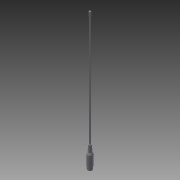
# Autodesk Inventor part: nagoya771
Saved by Autodesk Inventor 2014 (Build 180170000, 170)
## iProperties
Created: 2015-02-27
Part Number: nagoya771
Material: Generic
Document SubType Name: Modeling
Designer: Admin
Density: 1 g/cm^3
Appearance: Default
Author: Admin
Autodesk Inventor part; units mm, degrees
ref_plane "YZ Plane" through (0, 0, 0) normal (1, 0, 0) x (0, 1, 0)
ref_plane "XZ Plane" through (0, 0, 0) normal (0, 1, 0) x (-1, 0, 0)
ref_plane "XY Plane" through (0, 0, 0) normal (0, 0, 1) x (1, 0, 0)
sketch "Boceto1" plane through (0, 0, 0) normal (0, 0, 1) x (1, 0, 0)
  circle A0 centre (0, 0) radius 6.5
  dimension "d0" = 13
  constraints: 1 centre point, 1 coincident
  measures "d0" diameter of A0
extrude "Extrusión1" add sketch "Boceto1" along normal blind 8.25
sketch "Boceto2" plane through (0, 0, 8.25) normal (0, 0, 1) x (1, 0, 0)
  circle A0 centre (0, 0) radius 6.5 projected
  circle A1 centre (0, 0) radius 7.35
  dimension "d3" = 14.7
  constraints: 1 centre point, 1 coincident
  measures "d3" diameter of A1
extrude "Extrusión2" add sketch "Boceto2" along normal blind 29.75 contours A0 | A1
sketch "Boceto3" plane through (0, 0, 38) normal (0, 0, 1) x (1, 0, 0)
  circle A0 centre (0, 0) radius 7.35 projected
  circle A1 centre (0, 0) radius 5.65
  dimension "d6" = 11.3
  constraints: 1 centre point, 1 coincident
  measures "d6" diameter of A1
extrude "Extrusión3" add sketch "Boceto3" along normal blind 4.7 contours A1
sketch "Boceto4" plane through (0, 0, 0) normal (1, 0, 0) x (0, 1, 0)
  line L0 (5.65, 42.7) -> (-5.65, 42.7) projected
  line L1 (7.35, 38) -> (-7.35, 38) projected
  line L2 (5.65, 42.7) -> (7.35, 38)
  line L3 (5.65, 38) -> (5.65, 42.7)
  line L4 (0, 42.7) -> (0, 50.6655) construction
  point P0 (0, 0)
  constraints: 6 end point, 1 midpoint, 1 parallel, 1 perpendicular, 1 point on line
revolve "Revolución1" add sketch "Boceto4" angle 360 about axis through (0, 0, 42.7) along (0, 0, 1)
sketch "Boceto7" plane through (0, 0, 0) normal (1, 0, 0) x (0, 1, 0)
  line L0 (5.65, 42.7) -> (-5.65, 42.7) projected
  line L1 (0, 42.7) -> (4.95, 42.7) construction
  line L2 (0, 42.7) -> (0, 62.2)
  line L3 (0, 62.2) -> (3.9, 62.2)
  line L4 (3.9, 62.2) -> (4.95, 42.7)
  point P0 (0, 0)
  dimension "d13" = 4.95
  dimension "d14" = 19.5
  dimension "d15" = 3.9
  constraints: 8 end point, 2 perpendicular, 1 midpoint, 1 point on line
  measures "d13" distance of L1.start L1.end
  measures "d14" distance of L1.start L2.end
  measures "d15" distance of L2.end L3.end
revolve "Revolución2" add sketch "Boceto7" angle 360 about axis through (0, 0, 42.7) along (0, 0, 1)
sketch "Boceto8" plane through (0, 0, 62.2) normal (0, 0, 1) x (1, 0, 0)
  circle A0 centre (0, 0) radius 3.9 projected
  circle A1 centre (0, 0) radius 2.15
  dimension "d17" = 4.3
  constraints: 1 centre point, 1 coincident
  measures "d17" diameter of A1
extrude "Extrusión5" add sketch "Boceto8" along normal blind 82 contours A1
sketch "Boceto9" plane through (0, 0, 144.2) normal (0, 0, 1) x (1, 0, 0)
  circle A0 centre (0, 0) radius 2.15 projected
  circle A1 centre (0, 0) radius 1.95
  dimension "d20" = 3.9
  constraints: 1 centre point, 1 coincident
  measures "d20" diameter of A1
extrude "Extrusión6" add sketch "Boceto9" along normal blind 238 contours A1
sketch "Boceto10" plane through (0, 0, 382.2) normal (0, 0, 1) x (1, 0, 0)
  circle A0 centre (0, 0) radius 1.95 projected
  circle A1 centre (0, 0) radius 2.9
  dimension "d23" = 5.8
  constraints: 1 centre point, 1 coincident
  measures "d23" diameter of A1
extrude "Extrusión7" add sketch "Boceto10" along normal blind 13.4 contours A0 | A1
fillet "Empalme1" radius 2 1 edges at (-2.9, 0, 395.6)
fillet "Empalme2" radius 0.5 1 edges at (-2.9, 0, 382.2)
sketch "Boceto11" plane through (0, 0, 0) normal (0, 0, -1) x (-1, 0, 0)
  circle A0 centre (0, 0) radius 6.5 projected
  circle A1 centre (0, 0) radius 3.05
  dimension "d28" = 6.1
  constraints: 1 centre point, 1 coincident
  measures "d28" diameter of A1
hole "Hole1" at (0, 0, 0) direction (0, 0, 1) diameter 6.401 depth 15 thread size "5/16-18 UNC" class "1B" standard "ANSI Unified Screw Threads"
sketch "Boceto12" plane through (0, 0, 15) normal (0, 0, -1) x (-1, 0, 0)
  circle A0 centre (0, 0) radius 3.2005 projected
  circle A1 centre (0, 0) radius 0.25
  dimension "d36" = 0.5
  constraints: 1 centre point, 1 coincident
  measures "d36" diameter of A1
extrude "Extrusión8" cut sketch "Boceto12" against normal blind 10 contours A1
